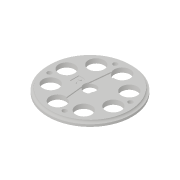
# Autodesk Inventor part: Right_Wheel_Disk
Saved by Autodesk Inventor 2019 (Build 230136000, 136)
## iProperties
Created: 2021-06-26
Part Number: Right_Wheel_Disk
Material: Generic
Document SubType Name: Modeling
Designer: Oudenas
Density: 1 g/cm^3
Appearance: Default
Author: Oudenas
Autodesk Inventor part; units mm, degrees
ref_plane "YZ Plane" through (0, 0, 0) normal (1, 0, 0) x (0, 1, 0)
ref_plane "XZ Plane" through (0, 0, 0) normal (0, 1, 0) x (-1, 0, 0)
ref_plane "XY Plane" through (0, 0, 0) normal (0, 0, 1) x (1, 0, 0)
sketch "Sketch1" plane through (0, 0, 0) normal (0, 1, 0) x (-1, 0, 0)
  circle A0 centre (0, 0) radius 28
  dimension "d0" = 56
  constraints: 1 centre point, 1 coincident
  measures "d0" diameter of A0
extrude "Extrusion1" add sketch "Sketch1" along normal blind 3
sketch "Sketch2" plane through (0, 3, 0) normal (0, 1, 0) x (1, 0, 0)
  circle A0 centre (0, 0) radius 3.5
  point P0 (3.4822, 0.3524)
  point P1 (-3.4822, 0.3524)
  point P2 (3.4822, -0.3524)
  point P3 (-3.4822, -0.3524)
  dimension "d53" = 7
  constraints: 4 point on circle, 1 centre point, 1 coincident
  measures "d53" diameter of A0
extrude "Extrusion2" cut sketch "Sketch2" against normal blind 3
sketch "Sketch5" plane through (0, 3, 0) normal (0, 1, 0) x (1, 0, 0)
  circle A0 centre (0, 0) radius 22.5 construction
  circle A1 centre (-5.0614, 21.9233) radius 1.5
  circle A2 centre (21.9233, 5.0614) radius 1.5
  circle A3 centre (5.0614, -21.9233) radius 1.5
  circle A4 centre (-21.9233, -5.0614) radius 1.5
  line L0 (0, 0) -> (-21.9233, -5.0614)
  line L1 (0, 0) -> (5.0614, -21.9233)
  line L2 (0, 0) -> (21.9233, 5.0614)
  line L3 (0, 0) -> (-5.0614, 21.9233)
  circle A5 centre (0, 0) radius 28 projected
  line L4 (0, 28) -> (0, -28) construction
  line L5 (28, 0) -> (-28, 0) construction
  dimension "d27" = 45
  dimension "d28" = 3
  dimension "d29" = 3
  dimension "d30" = 3
  dimension "d31" = 3
  dimension "d64" = 13
  dimension "d65" = 13
  dimension "d66" = 13
  dimension "d67" = 13
  constraints: 12 end point, 8 point on circle, 5 centre point, 3 point on line, 2 coincident, 1 perpendicular, 1 vertical
  measures "d27" diameter of A0
  measures "d28" diameter of A1
  measures "d29" diameter of A2
  measures "d30" diameter of A3
  measures "d31" diameter of A4
  measures "d64" angle of L3 L4
  measures "d65" angle of L0 L5
  measures "d66" angle of L1 L4
  measures "d67" angle of L2 L5
extrude "Extrusion5" cut sketch "Sketch5" against normal blind 3 contours A1 | A2 | A3 | A4
fillet "Fillet1" radius 1.5 1 edges at (28, 3, 0) inverted yes
sketch "Sketch6" plane through (0, 3, 0) normal (0, 1, 0) x (1, 0, 0)
  circle A0 centre (0, 0) radius 26.5 construction
  circle A1 centre (0, 0) radius 4.5 construction
  circle A2 centre (0, 0) radius 6.25 construction
  circle A3 centre (-21.9233, -5.0614) radius 1.5 construction
  circle A4 centre (0, 0) radius 22.5 construction
  circle A5 centre (0, 0) radius 18.75 construction
  circle A6 centre (0, 0) radius 26.5 construction
  circle A7 centre (-18.5183, 2.9386) radius 5.25
  dimension "d37" = 37.5
  dimension "d68" = 10.5
  dimension "d69" = 8
  constraints: 5 coincident, 4 centre point, 6 other
  measures "d68" diameter of A7
  measures "d69" vertical distance of A3.centre A7.centre
extrude "Extrusion7" cut sketch "Sketch6" against normal blind 3
pattern_circular "Circular Pattern2" count 8 over 360 about axis through (0, 3, 0) along (0, 1, 0) of "Extrusion7"
sketch "Sketch8" plane through (0, 3, 0) normal (0, 1, 0) x (1, 0, 0)
  circle A0 centre (0, 0) radius 3.5 construction
  line L0 (0, -15) -> (0, 15) construction
  arc A1 (-2, -15) -> (2, -15) centre (0, -15) ccw
  arc A2 (2, 15) -> (-2, 15) centre (0, 15) ccw
  circle A3 centre (0, 0) radius 3.5 projected
  line L1 (2, -15) -> (3.4822, -0.3524)
  line L2 (-2, -15) -> (-3.4822, -0.3524)
  line L3 (-2, 15) -> (-3.4822, 0.3524)
  line L4 (2, 15) -> (3.4822, 0.3524)
  dimension "d59" = 7
  dimension "d60" = 15
  dimension "d61" = 4
  constraints: 12 end point, 8 point on circle, 4 tangent, 3 centre point, 1 coincident, 1 midpoint, 1 vertical
  measures "d59" diameter of A0
  measures "d60" distance of A0.centre L0.end
  measures "d61" diameter of A2
extrude "Extrusion9" cut sketch "Sketch8" against normal blind 0.7 contours L2 A3 L1 A1 | L3 A2 L4 A3
sketch "Sketch9" plane through (0, 0, 0) normal (0, -1, 0) x (1, 0, 0)
  circle A0 centre (0, 0) radius 4
  dimension "d70" = 8
  constraints: 1 centre point, 1 coincident
  measures "d70" diameter of A0
extrude "Extrusion10" cut sketch "Sketch9" against normal blind 3
sketch "Sketch10" plane through (0, 3, 0) normal (0, 1, 0) x (1, 0, 0)
  line L0 (-11.4556, 3.3077) -> (-3.3452, 3.3077) construction
  line L1 (-3.3452, 3.3077) -> (-3.3452, -2.7923) construction
  line L2 (-3.3452, -2.7923) -> (-11.4556, -2.7923) construction
  line L3 (-11.4556, -2.7923) -> (-11.4556, 3.3077) construction
  spline S0 degree 2 poles (-5.264, -2.6033) (-5.264, -2.6548) (-5.3098, -2.7236) (-5.4759, -2.7751) (-5.8024, -2.7923) (-6.0831, -2.7923) knots 0 0 0 1 2 3 4 4 4
  spline S1 degree 2 poles (-6.0831, -2.7923) (-6.3179, -2.7923) (-6.6043, -2.7751) (-6.7647, -2.7236) (-6.8334, -2.6434) (-6.8563, -2.5861) knots 0 0 0 1 2 3 4 4 4
  line L4 (-6.8563, -2.5861) -> (-7.5093, -1.2286)
  spline S2 degree 2 poles (-7.5093, -1.2286) (-7.6238, -0.9995) (-7.8529, -0.6444) (-8.1279, -0.4039) (-8.4887, -0.2836) (-8.7235, -0.2836) knots 0 0 0 1 2 3 4 4 4
  line L5 (-8.7235, -0.2836) -> (-9.1818, -0.2836)
  line L6 (-9.1818, -0.2836) -> (-9.1818, -2.5918)
  spline S3 degree 2 poles (-9.1818, -2.5918) (-9.1818, -2.6434) (-9.2562, -2.7178) (-9.428, -2.7637) (-9.7087, -2.7923) (-9.9264, -2.7923) knots 0 0 0 1 2 3 4 4 4
  spline S4 degree 2 poles (-9.9264, -2.7923) (-10.1383, -2.7923) (-10.4247, -2.7637) (-10.5965, -2.7178) (-10.6652, -2.6434) (-10.6652, -2.5918) knots 0 0 0 1 2 3 4 4 4
  line L7 (-10.6652, -2.5918) -> (-10.6652, 2.9182)
  spline S5 degree 2 poles (-10.6652, 2.9182) (-10.6652, 3.1244) (-10.4075, 3.3077) (-10.2242, 3.3077) knots 0 0 0 1 2 2 2
  line L8 (-10.2242, 3.3077) -> (-8.3398, 3.3077)
  spline S6 degree 2 poles (-8.3398, 3.3077) (-8.0534, 3.3077) (-7.6811, 3.2905) (-7.5322, 3.2733) knots 0 0 0 1 2 2 2
  spline S7 degree 2 poles (-7.5322, 3.2733) (-7.0911, 3.2218) (-6.3866, 2.9698) (-5.8998, 2.5631) (-5.642, 2.0018) (-5.642, 1.6409) knots 0 0 0 1 2 3 4 4 4
  spline S8 degree 2 poles (-5.642, 1.6409) (-5.642, 1.3374) (-5.8253, 0.8333) (-6.1862, 0.4438) (-6.7131, 0.1517) (-7.051, 0.0601) knots 0 0 0 1 2 3 4 4 4
  spline S9 degree 2 poles (-7.051, 0.0601) (-6.8907, -0.0029) (-6.6043, -0.1919) (-6.3465, -0.4611) (-6.1232, -0.8048) (-6.0143, -1.0167) knots 0 0 0 1 2 3 4 4 4
  line L9 (-6.0143, -1.0167) -> (-5.4015, -2.2138)
  spline S10 degree 2 poles (-5.4015, -2.2138) (-5.3213, -2.3914) (-5.264, -2.5575) (-5.264, -2.6033) knots 0 0 0 1 2 2 2
  spline S11 degree 2 poles (-7.1713, 1.5149) (-7.1713, 1.8185) (-7.4978, 2.2309) (-7.8701, 2.3168) knots 0 0 0 1 2 2 2
  spline S12 degree 2 poles (-7.8701, 2.3168) (-7.9789, 2.3397) (-8.2653, 2.3683) (-8.5173, 2.3683) knots 0 0 0 1 2 2 2
  line L10 (-8.5173, 2.3683) -> (-9.1818, 2.3683)
  line L11 (-9.1818, 2.3683) -> (-9.1818, 0.6443)
  line L12 (-9.1818, 0.6443) -> (-8.4314, 0.6443)
  spline S13 degree 2 poles (-8.4314, 0.6443) (-8.1164, 0.6443) (-7.641, 0.7703) (-7.326, 0.9994) (-7.1713, 1.3202) (-7.1713, 1.5149) knots 0 0 0 1 2 3 4 4 4
  point P0 (0, 0)
  constraints: 2 other
extrude "Extrusion11" cut sketch "Sketch10" against normal blind 0.5
fillet "Fillet2" radius 0.4 4 edges at (-7.051, 2.75, -0.0601) (-9.1818, 2.75, -0.6443) (-9.1818, 2.75, 0.2836) (-9.1818, 2.75, -2.3683)
body "Solid1"
